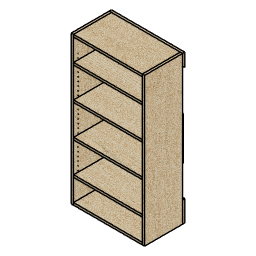
model (Autodesk Fusion 360 design; units mm, degrees)
Autodesk Fusion 360 part; units mm, degrees
note: some values were not read from the file. Chosen so that the rebuilt part matches the saved one: which bodies a step acts on; a side.
sketch "front" plane through (0, 0, 0) normal (0, 1, 0) x (1, 0, 0)
  line L0 (0, 0) -> (579, 0)
  line L1 (579, 0) -> (579, -1167)
  line L2 (579, -1167) -> (0, -1167)
  line L3 (0, -1167) -> (0, 0)
  line L4 (18, -18) -> (561, -18)
  line L5 (561, -18) -> (561, -1149)
  line L6 (561, -1149) -> (18, -1149)
  line L7 (18, -1149) -> (18, -18)
  line L8 (18, -1149) -> (18, -1167)
  line L9 (561, -1149) -> (561, -1167)
  line L10 (18, -18) -> (18, 0)
  line L11 (561, -18) -> (561, 0)
  line L12 (0, -753.5) -> (579, -753.5)
  line L13 (579, -413.5) -> (0, -413.5)
  line L14 (289.5, -753.5) -> (289.5, -1149) construction
  line L15 (289.5, -413.5) -> (289.5, -18) construction
  line L16 (0, -166) -> (579, -166)
  line L17 (0, -1062) -> (579, -1062)
  dimension "d1" = 1167
  dimension "d2" = 579
  dimension "d3" = 18
  dimension "d4" = 340
  dimension "d11" = 166
  dimension "d12" = 105
  constraint horizontal L0
  constraint vertical L1
  constraint horizontal L2
  constraint vertical L3
  constraint coincident L0.start L3.end
  constraint coincident L2 L8.end
  constraint perpendicular L2 L8
  constraint coincident L2 L9.end
  constraint perpendicular L2 L9
  constraint coincident L0 L10.end
  constraint perpendicular L0 L10
  constraint coincident L0 L11.end
  constraint perpendicular L0 L11
  constraint coincident L3 L12.start
  constraint coincident L1 L12.end
  constraint coincident L1 L13.start
  constraint coincident L3 L13.end
  constraint horizontal L13
  constraint horizontal L12
  constraint midpoint L12 L14.start
  constraint midpoint L6 L14.end
  constraint midpoint L13 L15.start
  constraint midpoint L4 L15.end
  constraint equal L14 L15
  constraint coincident L3 L16.start
  constraint coincident L1 L16.end
  constraint horizontal L16
  constraint coincident L3 L17.start
  constraint coincident L1 L17.end
  constraint horizontal L17
  measures "d1" distance of L0.start L2.end
  measures "d2" distance of L0.start L0.end
  measures "d4" distance of L12 L13
  measures "d11" distance of L0 L16
  measures "d12" distance of L2 L17
extrude "Extrude1" add sketch "front" along normal blind 6.35 contours L3 L7 L12 L13 | L5 L7 L12 L13 | L1 L5 L12 L13 makes body 1
extrude "Extrude2" add sketch "front" against normal blind 300 separate body contours L0 L3 L7 L10 L16 | L3 L7 L13 L16 | L0 L1 L5 L11 L16 | L3 L7 L12 L13 | L3 L7 L12 L17 | L1 L5 L13 L16 | L2 L3 L7 L8 L17 | L1 L5 L12 L13 | L1 L5 L12 L17 | L1 L2 L5 L9 L17 makes body 2 at (18, -100, 778) makes body 3 at (579, -100, 389)
extrude "Extrude3" add sketch "front" against normal blind 300 separate body contours L0 L4 L10 L11 | L2 L6 L8 L9 makes body 4 at (380, -100, 1149) makes body 5 at (199, -100, 0)
extrude "Extrude4" add sketch "front" along normal blind 18 separate body contours L0 L3 L7 L10 L16 | L0 L4 L10 L11 | L0 L1 L5 L11 L16 | L4 L5 L7 L16 | L2 L3 L7 L8 L17 | L5 L6 L7 L17 | L2 L6 L8 L9 | L1 L2 L5 L9 L17 makes body 6 at (193, 0, 1097) makes body 7 at (193, 0, 55.3333)
chamfer "Chamfer1" distance 18 angle 45 1 edges at (289.5, 0, 1062) on bodies 6
sketch "holes" plane through (18, 0, 0) normal (1, 0, 0) x (0, 1, 0)
  line L0 (0, 0) -> (0, 1167)
  line L1 (0, 1167) -> (-300, 1167)
  line L2 (-300, 1167) -> (-300, 0)
  line L3 (-300, 0) -> (0, 0)
  line L4 (-150, 0) -> (-150, 1167) construction
  line L5 (-263, 1167) -> (-263, 0) construction
  circle A0 centre (-263, 155) radius 3
  circle A1 centre (-263, 187) radius 3
  circle A2 centre (-263, 219) radius 3
  circle A3 centre (-263, 251) radius 3
  circle A4 centre (-263, 283) radius 3
  circle A5 centre (-263, 315) radius 3
  circle A6 centre (-263, 347) radius 3
  circle A7 centre (-263, 379) radius 3
  circle A8 centre (-263, 411) radius 3
  circle A9 centre (-263, 443) radius 3
  circle A10 centre (-263, 475) radius 3
  circle A11 centre (-263, 507) radius 3
  circle A12 centre (-263, 539) radius 3
  circle A13 centre (-263, 571) radius 3
  circle A14 centre (-263, 603) radius 3
  circle A15 centre (-263, 635) radius 3
  circle A16 centre (-263, 667) radius 3
  circle A17 centre (-263, 699) radius 3
  circle A18 centre (-263, 731) radius 3
  circle A19 centre (-263, 763) radius 3
  circle A20 centre (-263, 795) radius 3
  circle A21 centre (-263, 827) radius 3
  circle A22 centre (-263, 859) radius 3
  circle A23 centre (-263, 891) radius 3
  circle A24 centre (-263, 923) radius 3
  circle A25 centre (-263, 955) radius 3
  circle A26 centre (-263, 987) radius 3
  circle A27 centre (-263, 1019) radius 3
  circle A28 centre (-37, 475) radius 3
  circle A29 centre (-37, 859) radius 3
  circle A30 centre (-37, 155) radius 3
  circle A31 centre (-37, 315) radius 3
  circle A32 centre (-37, 507) radius 3
  circle A33 centre (-37, 1019) radius 3
  circle A34 centre (-37, 187) radius 3
  circle A35 centre (-37, 891) radius 3
  circle A36 centre (-37, 731) radius 3
  circle A37 centre (-37, 443) radius 3
  circle A38 centre (-37, 667) radius 3
  circle A39 centre (-37, 795) radius 3
  circle A40 centre (-37, 699) radius 3
  circle A41 centre (-37, 827) radius 3
  circle A42 centre (-37, 603) radius 3
  circle A43 centre (-37, 635) radius 3
  circle A44 centre (-37, 219) radius 3
  circle A45 centre (-37, 283) radius 3
  circle A46 centre (-37, 411) radius 3
  circle A47 centre (-37, 987) radius 3
  circle A48 centre (-37, 571) radius 3
  circle A49 centre (-37, 923) radius 3
  circle A50 centre (-37, 955) radius 3
  circle A51 centre (-37, 251) radius 3
  circle A52 centre (-37, 379) radius 3
  circle A53 centre (-37, 539) radius 3
  circle A54 centre (-37, 763) radius 3
  circle A55 centre (-37, 347) radius 3
  line L6 (-300, 208) -> (0, 208)
  line L7 (0, 190) -> (-300, 190)
  point P0 (-150, 208)
  dimension "d16" = 37
  dimension "d17" = 155
  dimension "d18" = 6
  dimension "d21" = 0
  dimension "d22" = 32
  dimension "d27" = 18
  constraint midpoint L3 L4.start
  constraint midpoint L1 L4.end
  constraint coincident L1 L5.start
  constraint coincident L3 L5.end
  constraint vertical L5
  constraint coincident L5 A0.centre
  constraint symmetric L4 A0 A30
  constraint symmetric L4 A1 A34
  constraint symmetric L4 A2 A44
  constraint symmetric L4 A3 A51
  constraint symmetric L4 A4 A45
  constraint symmetric L4 A5 A31
  constraint symmetric L4 A6 A55
  constraint symmetric L4 A7 A52
  constraint symmetric L4 A8 A46
  constraint symmetric L4 A9 A37
  constraint symmetric L4 A10 A28
  constraint symmetric L4 A11 A32
  constraint symmetric L4 A12 A53
  constraint symmetric L4 A13 A48
  constraint symmetric L4 A14 A42
  constraint symmetric L4 A15 A43
  constraint symmetric L4 A16 A38
  constraint symmetric L4 A17 A40
  constraint symmetric L4 A18 A36
  constraint symmetric L4 A19 A54
  constraint symmetric L4 A20 A39
  constraint symmetric L4 A21 A41
  constraint symmetric L4 A22 A29
  constraint symmetric L4 A23 A35
  constraint symmetric L4 A24 A49
  constraint symmetric L4 A25 A50
  constraint symmetric L4 A26 A47
  constraint symmetric L4 A27 A33
  constraint horizontal L6
  constraint horizontal L7
  constraint midpoint L6 P0
  constraint tangent A1 L7
  constraint coincident L0 L7.start
  constraint coincident L0 L6.end
  constraint coincident L2 L7.end
  measures "d16" distance of L2 L5
  measures "d17" distance of L5.end A0.centre
  measures "d18" diameter of A0
  measures "d27" distance of L6 L7
extrude "Extrude5" cut sketch "holes" along normal blind -10 and the other way up to surface (-553 mm away) contours A34 | A1 | A0 | A2 | A3 | A4 | A5 | A6 | A7 | A8 | A9 | A10 | A11 | A12 | A13 | A14 | A15 | A16 | A17 | A18 | A19 | A20 | A21 | A22 | A23 | A24 | A25 | A26 | A27 | A28 | A29 | A30 | A31 | A32 | A33 | A35 | A36 | A37 | A38 | A39 | A40 | A41 | A42 | A43 | A44 | A45 | A46 | A47 | A48 | A49 | A50 | A51 | A52 | A53 | A54 | A55 bodies 2 3
extrude "Extrude6" add sketch "holes" along normal up to surface (541 mm away) from surface at 1 separate body contours L0 L2 L6 L7 makes body 8
extrude "Extrude7" add sketch "holes" along normal blind 30 and the other way blind 10 separate body contours A34 | A1 makes body 9 at (34.6667, -262.627, 189.9767) makes body 10 at (21.3333, -34.1809, 188.0261)
chamfer "Chamfer2" distance 1 distance2 2 4 edges at (48, -265.797, 185.9152) (8, -265.797, 188.0848) (8, -39.797, 188.0848) (48, -39.797, 185.9152) measured on face at (48, -262.1435, 186.0323) measured on face at (8, -262.9253, 186.5923) measured on face at (8, -36.7225, 189.3424) measured on face at (48, -36.872, 184.6576) on bodies 9 10
ref_plane "WorkPlane1" through (289.5, -150, 583.5) normal (1, 0, 0) x (0, 0, 1)
mirror "Mirror1" about plane through (289.5, -150, 583.5) normal (1, 0, 0) of bodies 9 10 makes body 11 at (557, -261.6314, 189.6696) makes body 12 at (557, -34.1809, 188.0261)
pattern_linear "R-Pattern1" count 4 spacing 256 along (0, 0, 1) of bodies 9 10 12 8 11 makes body 13 at (199.3333, -200, 464) makes body 14 at (199.3333, -200, 720) makes body 15 at (199.3333, -200, 976) makes body 16 at (22, -261.2488, 445.4358) makes body 17 at (22, -260.3653, 700.4348) makes body 18 at (22, -260.3653, 956.4348) makes body 19 at (34, -38.9851, 445.2493) makes body 20 at (34, -34.4401, 700.5643) makes body 21 at (34, -34.4401, 956.5643) makes body 22 at (557, -261.2488, 445.4358) makes body 23 at (557, -260.3653, 700.4348) makes body 24 at (557, -260.3653, 956.4348) makes body 25 at (545, -38.9851, 445.2493) makes body 26 at (545, -34.4401, 700.5643) makes body 27 at (545, -34.4401, 956.5643)
equation "d5 = 1/4\""
equation "d42 = ( 32 * 8 ) * 1 mm"
